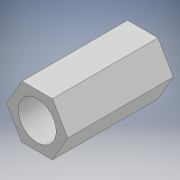
# Autodesk Inventor part: M3x10
Saved by Autodesk Inventor 2018 (Build 220112000, 112)
## iProperties
Created: 2017-10-04
Part Number: M3x10
Material: Generic
Document SubType Name: Modeling
Designer: leo2a
Density: 1 g/cm^3
Appearance: Default
Author: leo2a
Autodesk Inventor part; units mm, degrees
ref_plane "YZ Plane" through (0, 0, 0) normal (1, 0, 0) x (0, 1, 0)
ref_plane "XZ Plane" through (0, 0, 0) normal (0, 1, 0) x (-1, 0, 0)
ref_plane "XY Plane" through (0, 0, 0) normal (0, 0, 1) x (1, 0, 0)
sketch "Sketch3" plane through (0, 0, 0) normal (0, 1, 0) x (-1, 0, 0)
  line L0 (0, 0) -> (0, -2.5)
  line L1 (-1.4434, -2.5) -> (-2.8868, 0)
  line L2 (-2.8868, 0) -> (-1.4434, 2.5)
  line L3 (-1.4434, 2.5) -> (1.4434, 2.5)
  line L4 (1.4434, 2.5) -> (2.8868, 0)
  line L5 (2.8868, 0) -> (1.4434, -2.5)
  line L6 (1.4434, -2.5) -> (-1.4434, -2.5)
  dimension "d3" = 2.5
  constraints: 14 end point, 1 coincident, 1 midpoint, 1 vertical, 13 other
  measures "d3" distance of L0.start L0.end
extrude "Extrusion2" add sketch "Sketch3" along normal blind 10
sketch "Sketch4" plane through (0, 10, 0) normal (0, 1, 0) x (1, 0, 0)
  point P0 (0, 0)
  point P1 (0, 0)
  constraints: 1 coincident
hole "Hole1" at (0, 10, 0) direction (0, -1, 0) diameter 3.6 end through all clearance for "Socket Head Cap Screw ISO 4762" size "M3" standard "ISO"
body "Solid2"
